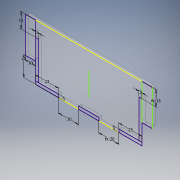
# Autodesk Inventor part: cham_back_v2
Saved by Autodesk Inventor 2017.2 (Build 212233000, 233)
## iProperties
Created: 2017-06-09
Part Number: cham_back_v2
Material: Generic
Document SubType Name: Modeling
Designer: SandeepSH
Density: 1 g/cm^3
Appearance: Polycarbonate - Clear
Author: SandeepSH
Autodesk Inventor part; units mm, degrees
ref_plane "YZ Plane" through (0, 0, 0) normal (1, 0, 0) x (0, 1, 0)
ref_plane "XZ Plane" through (0, 0, 0) normal (0, 1, 0) x (-1, 0, 0)
ref_plane "XY Plane" through (0, 0, 0) normal (0, 0, 1) x (1, 0, 0)
sketch "Sketch1" plane through (0, 0, 0) normal (0, 0, 1) x (1, 0, 0)
  line L0 (0, 0) -> (106, 0)
  line L1 (106, 0) -> (106, 55.5)
  line L2 (106, 55.5) -> (0, 55.5)
  line L3 (0, 55.5) -> (0, 0)
  dimension "d0" = 106
  dimension "d1" = 55.5
  constraints: 8 end point, 2 parallel, 1 horizontal, 1 perpendicular
  measures "d0" distance of L2.end L1.end
  measures "d1" distance of L1.end L0.end
extrude "Extrusion1" add sketch "Sketch1" along normal blind 3
sketch "Sketch2" plane through (0, 0, 3) normal (0, 0, 1) x (1, 0, 0)
  line L0 (106, 0) -> (106, 55.5) projected
  line L1 (106, 0) -> (83, 0)
  line L2 (83, 0) -> (83, 3)
  line L3 (83, 3) -> (106, 3)
  line L4 (106, 3) -> (106, 0)
  line L5 (0, 0) -> (106, 0) projected
  line L6 (0, 0) -> (23, 0)
  line L7 (23, 0) -> (23, 3)
  line L8 (23, 3) -> (0, 3)
  line L9 (0, 3) -> (0, 0)
  line L10 (43, 0) -> (63, 0)
  line L11 (63, 0) -> (63, 3)
  line L12 (63, 3) -> (43, 3)
  line L13 (43, 3) -> (43, 0)
  line L14 (0, 3) -> (3, 3)
  line L15 (3, 3) -> (3, 40.5)
  line L16 (3, 40.5) -> (0, 40.5)
  line L17 (0, 40.5) -> (0, 3)
  line L18 (106, 55.5) -> (0, 55.5) projected
  line L19 (106, 3) -> (103, 3)
  line L20 (103, 3) -> (103, 40.5)
  line L21 (103, 40.5) -> (106, 40.5)
  line L22 (106, 40.5) -> (106, 3)
  dimension "d4" = 23
  dimension "d5" = 3
  dimension "d6" = 23
  dimension "d7" = 3
  dimension "d8" = 20
  dimension "d9" = 20
  dimension "d10" = 3
  dimension "d11" = 15
  dimension "d12" = 3
  dimension "d13" = 15
  constraints: 40 end point, 10 parallel, 5 horizontal, 5 perpendicular, 2 point on line
  measures "d4" distance of L2.end L3.end
  measures "d5" distance of L1.end L2.end
  measures "d6" distance of L8.end L7.end
  measures "d7" distance of L7.end L6.end
  measures "d8" distance between parallel lines of L13 L7
  measures "d9" distance between parallel lines of L2 L11
  measures "d10" distance of L16.end L15.end
  measures "d11" distance between parallel lines of L16 L18
  measures "d12" distance of L20.end L21.end
  measures "d13" distance between parallel lines of L21 L18
extrude "Extrusion2" cut sketch "Sketch2" against normal through all
sketch "Sketch3" plane through (0, 0, 3) normal (0, 0, 1) x (1, 0, 0)
  line L0 (106, 55.5) -> (0, 55.5) projected
  line L1 (0, 55.5) -> (-10, 55.5)
  line L2 (-10, 55.5) -> (-10, 20)
  line L3 (-10, 20) -> (0, 20)
  line L4 (0, 20) -> (0, 55.5)
  line L5 (23, 0) -> (43, 0) projected
  line L6 (53, 38.2025) -> (53, 15.3086)
  line L7 (106, 55.5) -> (116, 55.5)
  line L8 (116, 55.5) -> (116, 20)
  line L9 (116, 20) -> (106, 20)
  line L10 (106, 20) -> (106, 55.5)
  point P0 (0, 0)
  dimension "d16" = 10
  dimension "d17" = 20
  constraints: 18 end point, 3 symmetric about line, 2 parallel, 1 horizontal, 1 perpendicular, 1 vertical
  measures "d16" distance of L3.end L2.end
  measures "d17" distance between parallel lines of L5 L3
extrude "Extrusion3" add sketch "Sketch3" against normal blind 3
fillet "Fillet1" radius 2 4 edges at (0, 20, 1.5) (116, 20, 1.5) (106, 20, 1.5) (-10, 20, 1.5) curvature continuous yes
fillet "Fillet2" radius 2 2 edges at (116, 55.5, 1.5) (-10, 55.5, 1.5) curvature continuous yes
equation "\"d9\" = d8"
equation "\"d13\" = d11"
body "Solid1"
